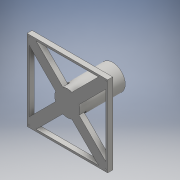
# Autodesk Inventor part: Motor housing for Lifting Platform
Saved by Autodesk Inventor 2016 (Build 200138000, 138)
## iProperties
Created: 2016-02-20
Part Number: Motor housing for Lifting Platform
Material: Generic
Document SubType Name: Modeling
Designer: Kenneth Daniel
Density: 1 g/cm^3
Appearance: Default
Author: Kenneth Daniel
Autodesk Inventor part; units mm, degrees
ref_plane "YZ Plane" through (0, 0, 0) normal (1, 0, 0) x (0, 1, 0)
ref_plane "XZ Plane" through (0, 0, 0) normal (0, 1, 0) x (-1, 0, 0)
ref_plane "XY Plane" through (0, 0, 0) normal (0, 0, 1) x (1, 0, 0)
sketch "Sketch1" plane through (0, 0, 0) normal (0, 1, 0) x (-1, 0, 0)
  line L0 (-40, 40) -> (-40, -40)
  line L1 (-40, -40) -> (40, -40)
  line L2 (40, -40) -> (40, 40)
  line L3 (40, 40) -> (-40, 40)
  line L4 (18.0792, 11.0081) -> (40, 32.9289)
  line L5 (11.6365, -4.5654) -> (40, -32.9289)
  line L6 (32.9289, -40) -> (4.5654, -11.6365)
  line L7 (-4.5654, 11.6365) -> (-32.9289, 40)
  line L8 (-11.6365, 4.5654) -> (-40, 32.9289)
  line L9 (32.9289, 40) -> (4.5654, 11.6365)
  line L10 (-11.6365, -4.5654) -> (-40, -32.9289)
  line L11 (-3.5355, 3.5355) -> (0, 0) construction
  line L12 (18.0792, 11.0081) -> (11.6365, 4.5654)
  line L13 (-4.5654, -11.6365) -> (-32.9289, -40)
  line L14 (30.8898, 37.9609) -> (-30.8898, 37.9609)
  line L15 (38, 30.9289) -> (38, -30.9289)
  line L16 (30.8898, -37.9609) -> (-30.8898, -37.9609)
  line L17 (-38.0969, -31.0259) -> (-38.0969, 31.0259)
  circle A0 centre (0, 0) radius 12.5
  point P0 (0, 0)
  dimension "d8" = 25
  dimension "d0" = 80
  dimension "d1" = 80
  dimension "d3" = 10
  dimension "d4" = 10
  dimension "d5" = 10
  dimension "d6" = 10
  dimension "d7" = 2
  dimension "d9" = 7.0711
  dimension "d10" = 7.0711
  dimension "d11" = 7.0711
  dimension "d12" = 7.0711
  dimension "d13" = 7.0711
  dimension "d14" = 7.0711
  dimension "d15" = 7.0711
  constraints: 36 end point, 17 point on line, 9 perpendicular, 8 parallel, 1 coincident, 1 vertical, 10 other
  measures "d0" distance of L0.start L0.end
  measures "d1" distance of L1.end L0.end
  measures "d3" distance between parallel lines of L9 L4
  measures "d4" distance between parallel lines of L6 L5
  measures "d5" distance between parallel lines of L10 L13
  measures "d6" distance between parallel lines of L7 L8
  measures "d7" distance between parallel lines of L2 L15
  measures "d9" distance of L9.start L2.end
  measures "d10" distance of L4.end L2.end
  measures "d11" distance of L1.end L5.end
  measures "d12" distance of L1.end L6.start
  measures "d13" distance of L13.end L0.end
  measures "d14" distance of L0.start L8.end
  measures "d15" distance of L7.end L0.start
extrude "Extrusion1" add sketch "Sketch1" along normal blind 5 contours L3 L7 A0 L8 L0 | L8 L17 L10 L0 | L3 L9 L14 L7 | L10 A0 L13 L1 L0 | L3 L2 L4 L12 A0 L9 | A0 | L13 L16 L6 L1 | L2 L5 L15 L4 | L6 A0 L5 L2 L1
sketch "Sketch2" plane through (0, 5, 0) normal (0, 1, 0) x (1, 0, 0)
  line L0 (-11.6365, -4.5654) -> (-38, -30.9289) projected
  line L1 (-38, -30.9289) -> (-38, 30.9289) projected
  line L2 (-38, 30.9289) -> (-11.6365, 4.5654) projected
  arc A0 (-11.6365, 4.5654) -> (-11.6365, -4.5654) centre (0, 0) ccw projected
  line L3 (-4.5654, 11.6365) -> (-30.8898, 37.9609) projected
  line L4 (-30.8898, 37.9609) -> (30.8898, 37.9609) projected
  line L5 (30.8898, 37.9609) -> (4.5654, 11.6365) projected
  arc A1 (4.5654, 11.6365) -> (-4.5654, 11.6365) centre (0, 0) ccw projected
  line L6 (11.6365, 4.5654) -> (38.0969, 31.0259) projected
  line L7 (38.0969, 31.0259) -> (38.0969, -31.0259) projected
  line L8 (38.0969, -31.0259) -> (11.6365, -4.5654) projected
  arc A2 (11.6365, -4.5654) -> (11.6365, 4.5654) centre (0, 0) ccw projected
  arc A3 (-4.5654, -11.6365) -> (4.5654, -11.6365) centre (0, 0) ccw projected
  line L9 (4.5654, -11.6365) -> (30.8898, -37.9609) projected
  line L10 (30.8898, -37.9609) -> (-30.8898, -37.9609) projected
  line L11 (-30.8898, -37.9609) -> (-4.5654, -11.6365) projected
  line L12 (-40, 40) -> (-40, -40) projected
  line L13 (-40, -40) -> (40, -40) projected
  line L14 (40, -40) -> (40, 40) projected
  line L15 (40, 40) -> (-40, 40) projected
  circle A4 centre (0, 0) radius 12.5
  point P0 (0, 0)
  constraints: 1 centre point, 1 coincident
extrude "Extrusion2" add sketch "Sketch2" along normal blind 40 contours A0 A4 A1 A2 A3
sketch "Sketch3" plane through (0, 45, 0) normal (0, 1, 0) x (1, 0, 0)
  circle A0 centre (0, 0) radius 11.5
  circle A1 centre (0, 0) radius 12.5 projected
  dimension "d20" = 1
  constraints: 1 centre point, 1 coincident
  measures "d20" radial gap between concentric circles of A1 A0
sketch "Sketch4" plane through (0, 5, 0) normal (0, 1, 0) x (1, 0, 0)
  line L0 (-40, 40) -> (-40, -40) projected
  line L1 (-40, -40) -> (40, -40) projected
  line L2 (40, -40) -> (40, 40) projected
  line L3 (40, 40) -> (-40, 40) projected
  arc A0 (-4.5654, 11.6365) -> (-11.6365, 4.5654) centre (0, 0) ccw projected
  line L4 (-4.5654, 11.6365) -> (-30.8898, 37.9609) projected
  line L5 (-30.8898, 37.9609) -> (30.8898, 37.9609) projected
  line L6 (30.8898, 37.9609) -> (4.5654, 11.6365) projected
  arc A1 (11.6365, 4.5654) -> (4.5654, 11.6365) centre (0, 0) ccw projected
  line L7 (11.6365, 4.5654) -> (38.0969, 31.0259) projected
  line L8 (38.0969, 31.0259) -> (38.0969, -31.0259) projected
  line L9 (38.0969, -31.0259) -> (11.6365, -4.5654) projected
  arc A2 (4.5654, -11.6365) -> (11.6365, -4.5654) centre (0, 0) ccw projected
  line L10 (4.5654, -11.6365) -> (30.8898, -37.9609) projected
  line L11 (30.8898, -37.9609) -> (-30.8898, -37.9609) projected
  line L12 (-30.8898, -37.9609) -> (-4.5654, -11.6365) projected
  arc A3 (-11.6365, -4.5654) -> (-4.5654, -11.6365) centre (0, 0) ccw projected
  line L13 (-11.6365, -4.5654) -> (-38, -30.9289) projected
  line L14 (-38, -30.9289) -> (-38, 30.9289) projected
  line L15 (-38, 30.9289) -> (-11.6365, 4.5654) projected
  line L16 (40, -40) -> (40, 40) construction
  line L17 (-40, 40) -> (40, -40) construction
  line L18 (40, -40) -> (-40, -40) construction
  line L19 (-40, -40) -> (40, 40) construction
  circle A4 centre (-38, 38) radius 1 construction
  circle A5 centre (-38, 38) radius 0.5
  line L20 (0, 42.5654) -> (0, -45.1181) construction
  line L21 (45.7517, 0) -> (-46.765, 0) construction
  circle A6 centre (38, 38) radius 0.5
  circle A7 centre (38, -38) radius 0.5
  circle A8 centre (-38, -38) radius 0.5
  point P0 (0, 0)
  dimension "d21" = 2
  dimension "d22" = 1
  constraints: 10 end point, 5 centre point, 3 symmetric about line, 1 coincident, 1 horizontal, 1 parallel, 1 point on line, 1 vertical, 3 other
  measures "d21" diameter of A4
  measures "d22" diameter of A5
extrude "Extrusion3" cut sketch "Sketch4" against normal blind 40 contours A5 | A6 | A7 | A8
sketch "Sketch5" plane through (0, 0, 0) normal (1, 0, 0) x (0, 1, 0)
  line L0 (0, -12.5) -> (45, -12.5) projected
  line L1 (5, -37.9609) -> (5, -11.6365) projected
  line L2 (0, -37.9609) -> (0, -11.6365) projected
  line L3 (0, -11.6365) -> (5, -11.6365) projected
  line L4 (0, -31.0259) -> (5, -31.0259) projected
  line L5 (5, -4.5654) -> (5, -31.0259) projected
  line L6 (0, -4.5654) -> (5, -4.5654) projected
  line L7 (0, -4.5654) -> (0, -31.0259) projected
  line L8 (0, 31.0259) -> (5, 31.0259) projected
  line L9 (0, 31.0259) -> (0, 4.5654) projected
  line L10 (0, 4.5654) -> (5, 4.5654) projected
  line L11 (5, 31.0259) -> (5, 4.5654) projected
  line L12 (5, 11.6365) -> (5, 4.5654) projected
  line L13 (0, 12.5) -> (45, 12.5) projected
  line L14 (5, -31.0259) -> (5, 31.0259) projected
  line L15 (5, 40) -> (5, -40) construction
  line L16 (5, -12.5) -> (7, -12.5) construction
  line L17 (7, -12.5) -> (7, 12.5) construction
  line L18 (7, -10.5) -> (5, -10.5)
  line L19 (7, 10.5) -> (5, 10.5)
  line L20 (7, -10.5) -> (7, 10.5)
  line L21 (5, -10.5) -> (5, 10.5)
  line L22 (7, 0) -> (5, 0)
  line L23 (-9, 0) -> (54, 0) projected
  point P0 (0, 0)
  dimension "d25" = 2
  dimension "d26" = 2
  dimension "d27" = 2
  constraints: 14 end point, 5 point on line, 3 perpendicular, 2 collinear, 2 midpoint, 4 other
  measures "d25" distance of L16.start L16.end
  measures "d26" distance of L16.end L18.start
  measures "d27" distance between parallel lines of L13 L19
revolve "Revolution1" cut sketch "Sketch5" angle 360 about axis through (0, -10, 0) along (0, 1, 0) contours L5 L14 L22 L20 L18
sketch "Sketch6" plane through (0, 5, 0) normal (0, 1, 0) x (1, 0, 0)
  circle A0 centre (0, 0) radius 12.5
  circle A1 centre (0, 0) radius 10.0217
  line L0 (11.6365, -4.5654) -> (0, 0)
  line L1 (0, 0) -> (4.6076, -11.6198)
  arc A2 (-4.5654, -11.6365) -> (4.5654, -11.6365) centre (0, 0) ccw projected
  line L2 (0, 0) -> (-4.5654, -11.6365)
  line L3 (-11.6365, -4.5654) -> (-38, -30.9289) projected
  line L4 (0, 0) -> (-11.6365, -4.5654)
  arc A3 (11.6365, -4.5654) -> (11.6365, 4.5654) centre (0, 0) ccw projected
  line L5 (0, 0) -> (11.6365, 4.5654)
  line L6 (11.6365, 4.5654) -> (0, 0)
  line L7 (0, 0) -> (4.5654, 11.6365)
  line L8 (0, 0) -> (-4.5654, 11.6365)
  line L9 (0, 0) -> (-11.6365, 4.5654)
  constraints: 18 end point, 5 point on circle, 3 perpendicular, 2 centre point, 2 coincident, 1 collinear
extrude "Extrusion4" cut sketch "Sketch6" along normal blind 2 contours A0 L1 A1 L0 | A1 L1 L0 | L8 A1 L9 A0 | L9 A1 L8
sketch "Sketch7" plane through (0, 5, 0) normal (0, 1, 0) x (1, 0, 0)
  arc A0 (11.6365, -4.5654) -> (11.6365, 4.5654) centre (0, 0) ccw projected
  arc A1 (4.5654, -11.6365) -> (11.6365, -4.5654) centre (0, 0) ccw
  arc A2 (-11.6365, -4.5654) -> (-4.5654, -11.6365) centre (0, 0) ccw
  arc A3 (11.6365, 4.5654) -> (4.5654, 11.6365) centre (0, 0) ccw
  arc A4 (-4.5654, 11.6365) -> (-11.6365, 4.5654) centre (0, 0) ccw
  line L0 (11.6365, -4.5654) -> (8.3603, -3.28)
  line L1 (-8.3603, 3.28) -> (-11.6365, 4.5654)
  line L2 (4.5654, -11.6365) -> (3.28, -8.3603)
  line L3 (-3.28, 8.3603) -> (-4.5654, 11.6365)
  line L4 (-4.5654, -11.6365) -> (-3.28, -8.3603)
  line L5 (3.28, 8.3603) -> (4.5654, 11.6365)
  line L6 (-11.6365, -4.5654) -> (-8.3603, -3.28)
  line L7 (8.3603, 3.28) -> (11.6365, 4.5654)
  arc A5 (3.28, -8.3603) -> (8.3603, -3.28) centre (0, 0) ccw
  arc A6 (-8.3603, -3.28) -> (-3.28, -8.3603) centre (0, 0) ccw
  arc A7 (8.3603, 3.28) -> (3.28, 8.3603) centre (0, 0) ccw
  arc A8 (-3.28, 8.3603) -> (-8.3603, 3.28) centre (0, 0) ccw
  dimension "d31" = 8.9807
  dimension "d32" = 3.2761
  dimension "d33" = 3.2761
  dimension "d34" = 3.2761
  constraints: 16 end point, 16 point on circle, 8 centre point, 5 concentric, 4 equal length, 2 coincident
  measures "d31" radius of A5
  measures "d32" horizontal distance of L0.start L0.end
  measures "d33" vertical distance of L2.start L2.end
  measures "d34" horizontal distance of L6.start L6.end
extrude "Extrusion5" cut sketch "Sketch7" along normal blind 2
extrude "Extrusion6" cut sketch "Sketch3" against normal blind 40 contours A0
sketch "Sketch8" plane through (0, 45, 0) normal (0, 1, 0) x (1, 0, 0)
  point P0 (0, 0)
body "Solid1"
